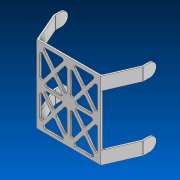
# Autodesk Inventor part: Elevator Tension
Saved by Autodesk Inventor 2022 (Build 260153000, 153)
## iProperties
Created: 2022-04-19
Part Number: Elevator Tension
Material: Generic
Document SubType Name: Modeling
Designer: score_nygvs6w
Density: 1 g/cm^3
Appearance: Default
Author: score_nygvs6w
Autodesk Inventor part; units mm, degrees
ref_plane "YZ Plane" through (0, 0, 0) normal (1, 0, 0) x (0, 1, 0)
ref_plane "XZ Plane" through (0, 0, 0) normal (0, 1, 0) x (-1, 0, 0)
ref_plane "XY Plane" through (0, 0, 0) normal (0, 0, 1) x (1, 0, 0)
sketch "Sketch1" plane through (0, 0, 0) normal (0, 0, 1) x (1, 0, 0)
  line L0 (63.5, 76.2) -> (-63.5, 76.2)
  line L1 (-63.5, 76.2) -> (-63.5, -76.2)
  line L2 (-63.5, -76.2) -> (63.5, -76.2)
  line L3 (63.5, -76.2) -> (63.5, 76.2)
  line L4 (63.5, 76.2) -> (-63.5, -76.2) construction
  line L5 (-63.5, 76.2) -> (63.5, -76.2) construction
  line L6 (-57.15, 69.85) -> (57.15, 69.85)
  line L7 (57.15, 69.85) -> (57.15, -69.85)
  line L8 (57.15, -69.85) -> (-57.15, -69.85)
  line L9 (-57.15, -69.85) -> (-57.15, 69.85)
  line L10 (-3.175, -69.85) -> (-3.175, 69.85)
  line L11 (3.175, 69.85) -> (3.175, -69.85)
  line L12 (0, 69.85) -> (0, -69.85) construction
  line L13 (-57.15, -69.85) -> (-3.175, 0) construction
  line L14 (-3.175, 0) -> (-57.15, 69.85) construction
  line L15 (3.175, 0) -> (57.15, 69.85) construction
  line L16 (3.175, 0) -> (57.15, -69.85) construction
  line L17 (3.175, -5.1926) -> (53.1375, -69.85)
  line L18 (57.15, -64.6574) -> (5.1812, 2.5963)
  line L19 (3.175, -5.1926) -> (57.15, 64.6574)
  line L20 (53.1375, 69.85) -> (3.175, 5.1926)
  line L21 (-3.175, 5.1926) -> (-53.1375, 69.85)
  line L22 (-57.15, 64.6574) -> (-3.175, -5.1926)
  line L23 (-3.175, 5.1926) -> (-57.15, -64.6574)
  line L24 (-53.1375, -69.85) -> (-3.175, -5.1926)
  line L25 (-57.15, 0) -> (-3.175, 69.85) construction
  line L26 (3.175, 69.85) -> (57.15, 0) construction
  line L27 (57.15, 0) -> (3.175, -69.85) construction
  line L28 (-3.175, -69.85) -> (-57.15, 0) construction
  line L29 (-5.6873, -71.7913) -> (-59.6623, -1.9413)
  line L30 (-59.6623, -1.9413) -> (-54.6377, 1.9413)
  line L31 (-54.6377, 1.9413) -> (-0.6627, -67.9087)
  line L32 (-0.6627, -67.9087) -> (-5.6873, -71.7913)
  line L33 (-5.6873, -71.7913) -> (-54.6377, 1.9413) construction
  line L34 (-59.6623, -1.9413) -> (-0.6627, -67.9087) construction
  line L35 (-54.6377, -1.9413) -> (-0.6627, 67.9087)
  line L36 (-0.6627, 67.9087) -> (-5.6873, 71.7913)
  line L37 (-5.6873, 71.7913) -> (-59.6623, 1.9413)
  line L38 (-59.6623, 1.9413) -> (-54.6377, -1.9413)
  line L39 (-54.6377, -1.9413) -> (-5.6873, 71.7913) construction
  line L40 (-0.6627, 67.9087) -> (-59.6623, 1.9413) construction
  line L41 (54.6377, -1.9413) -> (0.6627, 67.9087)
  line L42 (0.6627, 67.9087) -> (5.6873, 71.7913)
  line L43 (5.6873, 71.7913) -> (59.6623, 1.9413)
  line L44 (59.6623, 1.9413) -> (54.6377, -1.9413)
  line L45 (54.6377, -1.9413) -> (5.6873, 71.7913) construction
  line L46 (0.6627, 67.9087) -> (59.6623, 1.9413) construction
  line L47 (54.6377, 1.9413) -> (0.6627, -67.9087)
  line L48 (0.6627, -67.9087) -> (5.6873, -71.7913)
  line L49 (5.6873, -71.7913) -> (59.6623, -1.9413)
  line L50 (59.6623, -1.9413) -> (54.6377, 1.9413)
  line L51 (54.6377, 1.9413) -> (5.6873, -71.7913) construction
  line L52 (0.6627, -67.9087) -> (59.6623, -1.9413) construction
  line L53 (-3.175, 3.175) -> (-50.8115, 3.175)
  line L54 (-50.8115, 3.175) -> (-50.8115, -3.175)
  line L55 (-50.8115, -3.175) -> (-3.175, -3.175)
  line L56 (-3.175, -3.175) -> (-3.175, 3.175)
  line L57 (-3.175, 3.175) -> (-50.8115, -3.175) construction
  line L58 (-50.8115, 3.175) -> (-3.175, -3.175) construction
  line L59 (3.175, 3.175) -> (50.8, 3.175)
  line L60 (50.8, 3.175) -> (50.8, -3.175)
  line L61 (50.8, -3.175) -> (3.175, -3.175)
  line L62 (3.175, -3.175) -> (3.175, 3.175)
  line L63 (3.175, 3.175) -> (50.8, -3.175) construction
  line L64 (50.8, 3.175) -> (3.175, -3.175) construction
  point P0 (0, 0)
  point P1 (-30.1625, -34.925)
  point P2 (-30.1625, 34.925)
  point P3 (30.1625, 34.925)
  point P4 (30.1625, -34.925)
  point P5 (-26.9933, 0)
  point P6 (26.9875, 0)
  point P7 (-26.9933, 0)
  point P8 (0, 0)
  point P9 (26.9875, 0)
  point P10 (0, 0)
  point P11 (26.15, -34.925)
  point P12 (3.175, -64.6574)
  point P13 (-7.1875, 69.85)
  point P14 (-30.1625, 40.1176)
  point P15 (-9.6409, -3.175)
  point P16 (-30.1625, -29.7324)
  point P17 (-50.6841, -3.175)
  point P18 (26.15, 34.925)
  point P19 (3.175, 64.6574)
  point P20 (30.1625, 40.1176)
  point P21 (7.1875, 69.85)
  point P22 (30.1625, -40.1176)
  point P23 (7.1875, -69.85)
  point P24 (-26.15, -34.925)
  point P25 (-3.175, -64.6574)
  point P26 (-34.175, 34.925)
  point P27 (-57.15, 5.1926)
  point P28 (34.175, -34.925)
  point P29 (57.15, -5.1926)
  point P30 (30.1625, -29.7324)
  point P31 (9.6409, -3.175)
  point P32 (50.6841, -3.175)
  point P33 (34.175, 34.925)
  point P34 (57.15, 5.1926)
  point P35 (30.1625, 29.7324)
  point P36 (50.6841, 3.175)
  point P37 (9.6409, 3.175)
  point P38 (-50.6841, 3.175)
  point P39 (-30.1625, 29.7324)
  point P40 (-9.6409, 3.175)
  point P41 (-30.1625, -40.1176)
  point P42 (-7.1875, -69.85)
  point P43 (-34.175, -34.925)
  point P44 (-57.15, -5.1926)
  point P45 (-3.175, 64.6574)
  point P46 (-26.15, 34.925)
  dimension "d0" = 127
  dimension "d1" = 152.4
  dimension "d4" = 6.35
  dimension "d5" = 3.175
  dimension "d6" = 3.175
  dimension "d7" = 3.175
  dimension "d8" = 3.175
  dimension "d9" = 3.175
  dimension "d10" = 3.175
  constraints: 130 end point, 33 midpoint, 32 parallel, 20 point on line, 11 perpendicular, 5 equal length, 2 collinear, 2 horizontal, 2 horizontal alignment, 8 other
  measures "d0" distance of L0.start L0.end
  measures "d1" distance between parallel lines of L2 L0
  measures "d4" distance between parallel lines of L0 L6
  measures "d5" distance between parallel lines of L12 L10
  measures "d6" distance between parallel lines of L23 L13
  measures "d7" distance between parallel lines of L15 L20
  measures "d8" distance between parallel lines of L16 L18
  measures "d9" distance between parallel lines of L14 L22
  measures "d10" distance between parallel lines of L37 L25
extrude "Extrusion1" add sketch "Sketch1" along normal blind 3.175 contours L3 L2 L1 L0 | L6 L21 L37 L22 L9 | L37 L36 L6 | L6 L10 L35 L21 L37 | L21 L35 L22 L37 | L37 L22 L35 L53 L54 L31 L30 L9 | L9 L38 L37 | L36 L35 L10 | L6 L42 L41 L11 L47 L48 L8 L32 L31 L10 L35 L36 | L21 L23 L53 L22 L35 | L38 L35 L31 L54 L55 L23 L29 L9 | L9 L29 L30 | L30 L31 L35 L38 | L42 L43 L6 | L6 L43 L20 L41 L11 | L11 L41 L42 | L10 L53 L23 | L53 L23 L22 | L22 L23 L55 L31 L54 L35 L53 | L35 L54 L53 | L10 L55 L22 L23 L53 | L23 L29 L24 L8 L9 | L23 L31 L24 L29 | L35 L54 L31 | L22 L55 L23 | L6 L7 L19 L43 L20 | L43 L19 L41 L20 | L20 L41 L19 L59 L11 | L10 L22 L55 | L23 L55 L22 L24 L31 | L24 L31 L10 L8 L29 | L31 L55 L54 | L43 L7 L50 L47 L41 L60 L59 L19 | L59 L19 L61 L11 | L8 L32 L29 | L43 L44 L7 | L61 L19 L11 | L59 L41 L60 L47 L61 L18 L19 | L59 L60 L41 | L31 L32 L10 | L50 L49 L7 | L7 L49 L18 L47 L61 L60 L41 L44 | L44 L41 L47 L50 | L19 L61 L18 L47 L17 | L19 L18 L61 | L41 L47 L60 | L11 L47 L17 L49 L8 | L48 L47 L11 | L8 L49 L48 | L47 L18 L49 L17 | L60 L61 L47 | L7 L8 L17 L49 L18
fillet "Fillet1" radius 3.175 48 edges at (53.1375, -69.85, 1.5875) (57.15, -64.6574, 1.5875) (34.175, -34.925, 1.5875) (57.15, -5.1926, 1.5875) (50.6841, -3.175, 1.5875) (50.6841, 3.175, 1.5875) (57.15, 5.1926, 1.5875) (30.1625, -40.1176, 1.5875) (26.15, -34.925, 1.5875) (30.1625, -29.7324, 1.5875) (7.1875, -69.85, 1.5875) (3.175, -64.6574, 1.5875) (3.175, -5.1926, 1.5875) (9.6409, -3.175, 1.5875) (-3.175, -64.6574, 1.5875) (-7.1875, -69.85, 1.5875) (-30.1625, -40.1176, 1.5875) (-53.1375, -69.85, 1.5875) (-57.15, -64.6574, 1.5875) (-34.175, -34.925, 1.5875) (-30.1625, -29.7324, 1.5875) (-26.15, -34.925, 1.5875) (-3.175, -5.1926, 1.5875) (-9.6409, -3.175, 1.5875) (-50.6841, -3.175, 1.5875) (-57.15, -5.1926, 1.5875) (-50.6841, 3.175, 1.5875) (-57.15, 5.1926, 1.5875) (-9.6409, 3.175, 1.5875) (-3.175, 5.1926, 1.5875) (3.175, 5.1926, 1.5875) (9.6409, 3.175, 1.5875) (30.1625, 29.7324, 1.5875) (34.175, 34.925, 1.5875) (26.15, 34.925, 1.5875) (30.1625, 40.1176, 1.5875) (57.15, 64.6574, 1.5875) (53.1375, 69.85, 1.5875) (7.1875, 69.85, 1.5875) (3.175, 64.6574, 1.5875) (-26.15, 34.925, 1.5875) (-3.175, 64.6574, 1.5875) (-7.1875, 69.85, 1.5875) (-53.1375, 69.85, 1.5875) (-30.1625, 40.1176, 1.5875) (-30.1625, 29.7324, 1.5875) (-34.175, 34.925, 1.5875) (-57.15, 64.6574, 1.5875)
sketch "Sketch2" plane through (-63.5, 76.2, 0) normal (0, 1, 0) x (1, 0, 0)
  line L0 (-25.4, 80.9625) -> (-22.225, 80.9625)
  line L1 (-22.225, 80.9625) -> (-22.225, 55.5625)
  line L2 (-22.225, 55.5625) -> (-25.4, 55.5625)
  line L3 (-25.4, 55.5625) -> (-25.4, 80.9625)
  line L4 (152.4, 80.9625) -> (149.225, 80.9625)
  line L5 (149.225, 80.9625) -> (149.225, 55.5625)
  line L6 (149.225, 55.5625) -> (152.4, 55.5625)
  line L7 (152.4, 55.5625) -> (152.4, 80.9625)
  line L8 (127, -3.175) -> (0, -3.175) projected
  line L9 (63.5, 0) -> (63.5, 80.9625) construction
  line L10 (127, 0) -> (0, 0) projected
  line L11 (0, 0) -> (0, -3.175) projected
  line L12 (127, -3.175) -> (0, -3.175) projected
  line L13 (127, 0) -> (127, -3.175) projected
  line L14 (0, 0) -> (0, -3.175) projected
  line L15 (0, -3.175) -> (-25.4, 55.5625)
  line L16 (0, 0) -> (127, 0) projected
  line L17 (2.0862, 0) -> (-22.225, 56.2196)
  line L18 (127, 0) -> (127, -3.175) projected
  line L19 (127, -3.175) -> (152.4, 55.5625)
  line L20 (149.225, 56.2196) -> (124.9138, 0)
  point P0 (2.0862, 0)
  dimension "d12" = 25.4
  dimension "d13" = 58.7375
  dimension "d14" = 3.175
  dimension "d15" = 177.8
  dimension "d16" = 3.175
  dimension "d17" = 3.175
  constraints: 26 end point, 6 parallel, 5 point on line, 2 equal length, 2 horizontal, 2 perpendicular, 1 collinear, 1 vertical, 1 other
  measures "d12" distance of L0.end L1.end
  measures "d13" distance between parallel lines of L2 L8
  measures "d14" distance between parallel lines of L3 L1
  measures "d15" distance between parallel lines of L7 L3
  measures "d16" distance between parallel lines of L15 L17
  measures "d17" distance between parallel lines of L19 L20
extrude "Extrusion2" add sketch "Sketch2" against normal blind 25.4 contours L0 L1 L2 L3 | L2 L1 L17 L10 L11 L15 | L13 L10 L20 L5 L6 L19 | L6 L5 L4 L7
fillet "Fillet2" radius 3.81 8 edges at (-61.4138, 63.5, 0) (-85.725, 63.5, -56.2196) (61.4138, 63.5, 0) (62.4569, 50.8, 0) (-62.4569, 50.8, 0) (85.725, 63.5, -56.2196) (88.9, 63.5, -55.5625) (-88.9, 63.5, -55.5625)
fillet "Fillet2" radius 1.27 2 edges at (63.5, 50.8, 1.5875) (-63.5, 50.8, 1.5875)
fillet "Fillet3" radius 12.7 4 edges at (87.3125, 50.8, -80.9625) (87.3125, 76.2, -80.9625) (-87.3125, 50.8, -80.9625) (-87.3125, 76.2, -80.9625)
mirror "Mirror1" about plane through (0, 0, 0) normal (0, 1, 0) of "Fillet3", "Fillet2", "Extrusion2"
equation "\"d6\" = d5"
equation "\"d7\" = d5"
equation "\"d8\" = d7"
equation "\"d9\" = d5"
equation "\"d10\" = d5"
body "Solid1"
